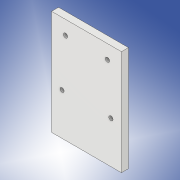
# Autodesk Inventor part: GA006
Saved by Autodesk Inventor 2017 SP1 (Build 210196100, 196)
## iProperties
Created: 2017-06-20
Part Number: GA006
Material: ABS Plastic
Document SubType Name: Modeling
Designer: zallen
Density: 1.06 g/cm^3
Appearance: CR White
Author: zallen
Autodesk Inventor part; units mm, degrees
ref_plane "YZ Plane" through (0, 0, 0) normal (1, 0, 0) x (0, 1, 0)
ref_plane "XZ Plane" through (0, 0, 0) normal (0, 1, 0) x (-1, 0, 0)
ref_plane "XY Plane" through (0, 0, 0) normal (0, 0, 1) x (1, 0, 0)
sketch "Sketch1" plane through (0, 0, 0) normal (0, 0, 1) x (1, 0, 0)
  line L0 (0, 0) -> (50, 0)
  line L1 (50, 0) -> (50, 75)
  line L2 (50, 75) -> (0, 75)
  line L3 (0, 75) -> (0, 0)
  line L4 (10, 65) -> (40, 65) construction
  line L5 (40, 65) -> (42.5, 30) construction
  line L6 (42.5, 30) -> (7.5, 30) construction
  line L7 (7.5, 30) -> (10, 65) construction
  line L8 (8.75, 47.5) -> (41.25, 47.5) construction
  line L9 (25, 65) -> (25, 30) construction
  circle A0 centre (10, 65) radius 1.5
  circle A1 centre (7.5, 30) radius 1.5
  circle A2 centre (42.5, 30) radius 1.5
  circle A3 centre (40, 65) radius 1.5
  point P0 (25, 75)
  dimension "d0" = 50
  dimension "d1" = 75
  dimension "d2" = 35
  dimension "d4" = 3
  dimension "d5" = 3
  dimension "d6" = 3
  dimension "d7" = 3
  dimension "d8" = 10
  dimension "d11" = 30
  dimension "d12" = 35
  constraints: 20 end point, 5 midpoint, 4 centre point, 4 coincident, 3 parallel, 2 horizontal, 1 perpendicular, 1 vertical, 1 vertical alignment
  measures "d0" distance of L2.end L1.end
  measures "d1" distance of L1.end L0.end
  measures "d2" distance of L5.end L6.end
  measures "d4" diameter of A0
  measures "d5" diameter of A1
  measures "d6" diameter of A2
  measures "d7" diameter of A3
  measures "d8" distance of point (25, 75) L9.start
  measures "d11" distance of L4.start L4.end
  measures "d12" distance between parallel lines of L6 L4
extrude "Extrusion1" add sketch "Sketch1" along normal blind 5
body "Solid1"
